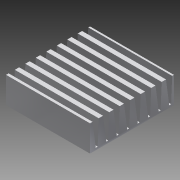
# Autodesk Inventor part: HeatSink60
Saved by Autodesk Inventor 2014 (Build 180170000, 170)
## iProperties
Created: 2015-04-18
Part Number: HeatSink60
Material: Generic
Document SubType Name: Modeling
Designer: Owner
Density: 1 g/cm^3
Appearance: Aluminum - Polished
Author: Owner
Autodesk Inventor part; units mm, degrees
ref_plane "YZ Plane" through (0, 0, 0) normal (1, 0, 0) x (0, 1, 0)
ref_plane "XZ Plane" through (0, 0, 0) normal (0, 1, 0) x (-1, 0, 0)
ref_plane "XY Plane" through (0, 0, 0) normal (0, 0, 1) x (1, 0, 0)
sketch "Sketch1" plane through (0, 0, 0) normal (0, 1, 0) x (-1, 0, 0)
  line L0 (-47.5907, 29.7008) -> (54.0093, 29.7008)
  line L1 (54.0093, 29.7008) -> (54.0093, -71.8992)
  line L2 (54.0093, -71.8992) -> (-47.5907, -71.8992)
  line L3 (-47.5907, -71.8992) -> (-47.5907, 29.7008)
  point P0 (0, 0)
  dimension "d0" = 101.6
  dimension "d1" = 101.6
  constraints: 8 end point, 2 parallel, 1 horizontal, 1 perpendicular
  measures "d0" distance of L0.start L0.end
  measures "d1" distance of L0.end L1.end
extrude "Extrusion1" add sketch "Sketch1" along normal blind 31.75
sketch "Sketch2" plane through (47.5907, 0, 29.7008) normal (1, 0, 0) x (0, 0, -1)
  line L0 (0, 31.75) -> (101.6, 31.75) projected
  line L1 (2.6537, 35.2563) -> (7.0386, 2.4572)
  line L2 (7.0386, 2.4572) -> (9.3017, 2.7597)
  line L3 (9.3017, 2.7597) -> (10.7219, 35.2563)
  line L4 (10.7219, 35.2563) -> (2.6537, 35.2563)
  point P0 (29.7008, 0)
  constraints: 8 end point, 1 parallel, 1 perpendicular
extrude "Extrusion2" cut sketch "Sketch2" against normal up to next
pattern_linear "Rectangular Pattern1" count 8 spacing 12.7 along (0, 0, -1) of "Extrusion2"
body "Solid1"
